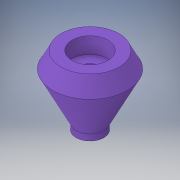
# Autodesk Inventor part: Train smoke stack
Saved by Autodesk Inventor 2017.1 (Build 211199000, 199)
## iProperties
Created: 2017-04-26
Part Number: Train smoke stack
Material: ABS Plastic
Document SubType Name: Modeling
Designer: 196918
Density: 1.06 g/cm^3
Appearance: Violet
Author: 196918
Autodesk Inventor part; units mm, degrees
ref_plane "YZ Plane" through (0, 0, 0) normal (1, 0, 0) x (0, 1, 0)
ref_plane "XZ Plane" through (0, 0, 0) normal (0, 1, 0) x (-1, 0, 0)
ref_plane "XY Plane" through (0, 0, 0) normal (0, 0, 1) x (1, 0, 0)
sketch "Sketch1" plane through (0, 0, 0) normal (1, 0, 0) x (0, 1, 0)
  line L0 (1.947, 4.4699) -> (0, 4.4699)
  line L1 (0, 4.4699) -> (0, 0)
  line L2 (0, 0) -> (1.947, 0)
  line L3 (1.947, 0) -> (1.947, 4.4699)
  constraints: 8 end point, 2 parallel, 1 horizontal, 1 perpendicular
sketch "Sketch2" plane through (0, 0, 0) normal (1, 0, 0) x (0, 1, 0)
  line L0 (1.947, 0) -> (1.947, 4.4699) projected
  line L1 (0, 0) -> (1.947, 0) projected
  line L2 (1.947, 4.4699) -> (0, 4.4699) projected
  line L3 (16.9602, -1.2877) -> (22.1681, -1.2877)
  line L4 (22.1681, -1.2877) -> (22.1681, -4.8754)
  line L5 (22.1681, -4.8754) -> (16.9602, -7.5373)
  line L6 (16.9602, -7.5373) -> (1.947, 0)
  line L7 (1.947, 2.235) -> (16.9602, 2.235)
  line L8 (16.9602, 2.235) -> (16.9602, -1.2877)
  line L9 (1.947, 4.4699) -> (5.6822, 4.4699)
  constraints: 14 end point, 2 horizontal, 2 perpendicular, 1 midpoint
sketch "Sketch3" plane through (0, 0, 0) normal (1, 0, 0) x (0, 1, 0)
  point P0 (0, 0)
revolve "Revolution1" add sketch "Sketch2" angle 360 about axis through (0, 1.947, 4.4699) along (0, 1, 0)
revolve "Revolution2" add sketch "Sketch1" angle 360 about axis through (0, 1.947, 4.4699) along (0, -1, 0)
body "Solid1"
